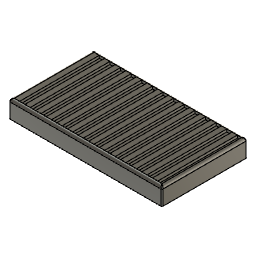
IFEI Clear 0.5mm-0.25 F4 v1 (Autodesk Fusion 360 design; units mm, degrees)
Autodesk Fusion 360 part; units mm, degrees
sketch "Sketch1" plane through (0, 0, 0) normal (0, 0, 1) x (1, 0, 0) in component "Clear"
  line L0 (-0.4, -0.5) -> (13.8, -0.5)
  line L1 (13.9, -0.4) -> (13.9, 7.4)
  line L2 (13.8, 7.5) -> (-0.4, 7.5)
  line L3 (-0.5, 7.4) -> (-0.5, -0.4)
  arc A0 (-0.4, 7.5) -> (-0.5, 7.4) centre (-0.4, 7.4) ccw
  arc A1 (-0.5, -0.4) -> (-0.4, -0.5) centre (-0.4, -0.4) ccw
  arc A2 (13.8, -0.5) -> (13.9, -0.4) centre (13.8, -0.4) ccw
  arc A3 (13.9, 7.4) -> (13.8, 7.5) centre (13.8, 7.4) ccw
  dimension "d4" = 0.1
  dimension "d5" = 0.1
  dimension "d6" = 0.1
  dimension "d7" = 0.1
  constraint tangent L2 A0
  constraint tangent L3 A0
  constraint tangent L3 A1
  constraint tangent L0 A1
  constraint tangent L0 A2
  constraint tangent L1 A2
  constraint tangent L2 A3
  constraint tangent L1 A3
  measures "d4" radius of A0
  measures "d5" radius of A1
  measures "d6" radius of A2
  measures "d7" radius of A3
extrude "Extrude1" add sketch "Sketch1" along normal blind 1.9 in component "Clear"
fillet "Fillet1" radius 0.25 1 faces at (4.3333, 4.8333, 1.9) in component "Clear"
sketch "Sketch1 (2)" plane through (0, 0, 1.9) normal (0, 0, 1) x (-1, 0, 0)
  line L0 (-13.65, 0.25) -> (-13.65, -7.25)
  line L1 (-13.65, -7.25) -> (0.25, -7.25)
  line L2 (0.25, -7.25) -> (0.25, 0.25)
  line L3 (0.25, 0.25) -> (-13.65, 0.25)
  line L4 (0.25, -7.25) -> (-0.25, -7.25) construction
  line L5 (-0.25, -7.25) -> (-0.75, -7.25)
  line L6 (-0.75, -7.25) -> (-0.75, 0.25)
  line L7 (-0.75, 0.25) -> (-0.25, 0.25)
  line L8 (-0.25, 0.25) -> (-0.25, -7.25)
  line L9 (-0.75, -7.25) -> (-1.25, -7.25) construction
  line L10 (-1.75, 0.25) -> (-1.25, 0.25)
  line L11 (-1.75, -7.25) -> (-2.25, -7.25) construction
  line L12 (-1.25, 0.25) -> (-1.25, -7.25)
  line L13 (-1.75, -7.25) -> (-1.75, 0.25)
  line L14 (-1.25, -7.25) -> (-1.75, -7.25)
  line L15 (-3.25, -7.25) -> (-3.75, -7.25)
  line L16 (-2.25, 0.25) -> (-2.25, -7.25)
  line L17 (-2.25, -7.25) -> (-2.75, -7.25)
  line L18 (-3.25, 0.25) -> (-3.25, -7.25)
  line L19 (-3.75, -7.25) -> (-3.75, 0.25)
  line L20 (-3.75, -7.25) -> (-4.25, -7.25) construction
  line L21 (-2.75, 0.25) -> (-2.25, 0.25)
  line L22 (-2.75, -7.25) -> (-2.75, 0.25)
  line L23 (-2.75, -7.25) -> (-3.25, -7.25) construction
  line L24 (-3.75, 0.25) -> (-3.25, 0.25)
  line L25 (-6.75, 0.25) -> (-6.25, 0.25)
  line L26 (-5.25, 0.25) -> (-5.25, -7.25)
  line L27 (-7.75, 0.25) -> (-7.25, 0.25)
  line L28 (-5.75, 0.25) -> (-5.25, 0.25)
  line L29 (-5.25, -7.25) -> (-5.75, -7.25)
  line L30 (-6.75, -7.25) -> (-6.75, 0.25)
  line L31 (-4.75, -7.25) -> (-4.75, 0.25)
  line L32 (-4.75, -7.25) -> (-5.25, -7.25) construction
  line L33 (-6.25, 0.25) -> (-6.25, -7.25)
  line L34 (-4.75, 0.25) -> (-4.25, 0.25)
  line L35 (-7.75, -7.25) -> (-8.25, -7.25) construction
  line L36 (-5.75, -7.25) -> (-6.25, -7.25) construction
  line L37 (-4.25, 0.25) -> (-4.25, -7.25)
  line L38 (-5.75, -7.25) -> (-5.75, 0.25)
  line L39 (-7.25, -7.25) -> (-7.75, -7.25)
  line L40 (-6.75, -7.25) -> (-7.25, -7.25) construction
  line L41 (-7.75, -7.25) -> (-7.75, 0.25)
  line L42 (-7.25, 0.25) -> (-7.25, -7.25)
  line L43 (-6.25, -7.25) -> (-6.75, -7.25)
  line L44 (-4.25, -7.25) -> (-4.75, -7.25)
  line L45 (-12.75, 0.25) -> (-12.25, 0.25)
  line L46 (-13.75, 0.25) -> (-13.25, 0.25)
  line L47 (-8.75, -7.25) -> (-8.75, 0.25)
  line L48 (-13.25, 0.25) -> (-13.25, -7.25)
  line L49 (-8.75, 0.25) -> (-8.25, 0.25)
  line L50 (-9.75, -7.25) -> (-10.25, -7.25) construction
  line L51 (-8.25, 0.25) -> (-8.25, -7.25)
  line L52 (-8.25, -7.25) -> (-8.75, -7.25)
  line L53 (-8.75, -7.25) -> (-9.25, -7.25) construction
  line L54 (-9.25, 0.25) -> (-9.25, -7.25)
  line L55 (-10.75, -7.25) -> (-10.75, 0.25)
  line L56 (-10.75, 0.25) -> (-10.25, 0.25)
  line L57 (-10.75, -7.25) -> (-11.25, -7.25) construction
  line L58 (-9.75, 0.25) -> (-9.25, 0.25)
  line L59 (-11.75, 0.25) -> (-11.25, 0.25)
  line L60 (-11.75, -7.25) -> (-12.25, -7.25) construction
  line L61 (-13.25, -7.25) -> (-13.75, -7.25)
  line L62 (-12.25, 0.25) -> (-12.25, -7.25)
  line L63 (-14.75, -7.25) -> (-15.25, -7.25) construction
  line L64 (-13.75, -7.25) -> (-14.25, -7.25) construction
  line L65 (-12.75, -7.25) -> (-13.25, -7.25) construction
  line L66 (-10.25, -7.25) -> (-10.75, -7.25)
  line L67 (-12.25, -7.25) -> (-12.75, -7.25)
  line L68 (-12.75, -7.25) -> (-12.75, 0.25)
  line L69 (-11.25, 0.25) -> (-11.25, -7.25)
  line L70 (-13.75, -7.25) -> (-13.75, 0.25)
  line L71 (-11.75, -7.25) -> (-11.75, 0.25)
  line L72 (-11.25, -7.25) -> (-11.75, -7.25)
  line L73 (-9.75, -7.25) -> (-9.75, 0.25)
  line L74 (-10.25, 0.25) -> (-10.25, -7.25)
  line L75 (-9.25, -7.25) -> (-9.75, -7.25)
  point P0 (-8.25, -7.25)
  dimension "d11" = 0.5
  dimension "d12" = 0.5
  dimension "d13" = 0.5
  dimension "d14" = 0.5
  dimension "d15" = 0.5
  dimension "d16" = 0.5
  dimension "d17" = 0.5
  dimension "d18" = 0.5
  dimension "d19" = 0.5
  dimension "d20" = 0.5
  dimension "d21" = 0.5
  dimension "d22" = 0.5
  dimension "d23" = 0.5
  dimension "d24" = 0.5
  dimension "d25" = 0.5
  dimension "d26" = 0.5
  dimension "d27" = 0.5
  dimension "d28" = 0.5
  dimension "d29" = 0.5
  dimension "d30" = 0.5
  dimension "d31" = 0.5
  dimension "d32" = 0.5
  dimension "d33" = 0.5
  dimension "d34" = 0.5
  dimension "d35" = 0.5
  dimension "d36" = 0.5
  dimension "d37" = 0.5
  dimension "d38" = 0.5
  dimension "d39" = 0.5
  dimension "d41" = 0.5
  constraint coincident L1.end L2.start
  constraint perpendicular L2 L4
  constraint horizontal L5
  constraint vertical L6
  constraint horizontal L7
  constraint vertical L8
  constraint coincident L3 L6.end
  constraint perpendicular L6 L9
  constraint horizontal L14
  constraint vertical L13
  constraint horizontal L10
  constraint vertical L12
  constraint perpendicular L11 L13
  constraint horizontal L17
  constraint vertical L22
  constraint horizontal L21
  constraint vertical L16
  constraint perpendicular L22 L23
  constraint horizontal L15
  constraint vertical L19
  constraint horizontal L24
  constraint vertical L18
  constraint perpendicular L19 L20
  constraint horizontal L44
  constraint vertical L31
  constraint horizontal L34
  constraint vertical L37
  constraint perpendicular L31 L32
  constraint horizontal L29
  constraint vertical L38
  constraint horizontal L28
  constraint vertical L26
  constraint perpendicular L36 L38
  constraint horizontal L43
  constraint vertical L30
  constraint horizontal L25
  constraint vertical L33
  constraint perpendicular L30 L40
  constraint horizontal L39
  constraint vertical L41
  constraint horizontal L27
  constraint vertical L42
  constraint perpendicular L35 L41
  constraint horizontal L52
  constraint vertical L47
  constraint horizontal L49
  constraint vertical L51
  constraint perpendicular L47 L53
  constraint horizontal L75
  constraint vertical L73
  constraint horizontal L58
  constraint vertical L54
  constraint perpendicular L50 L73
  constraint horizontal L66
  constraint vertical L55
  constraint horizontal L56
  constraint vertical L74
  constraint perpendicular L55 L57
  constraint horizontal L72
  constraint vertical L71
  constraint horizontal L59
  constraint vertical L69
  constraint perpendicular L60 L71
  constraint horizontal L67
  constraint vertical L68
  constraint horizontal L45
  constraint vertical L62
  constraint perpendicular L65 L68
  constraint horizontal L61
  constraint vertical L70
  constraint horizontal L46
  constraint vertical L48
  constraint perpendicular L64 L70
  measures "d11" distance of L1.end L4.end
  measures "d12" distance of L4.end L5.end
  measures "d13" distance of L5.end L9.end
  measures "d14" distance of L11.start L9.end
  measures "d15" distance of L11.start L11.end
  measures "d16" distance of L17.end L11.end
  measures "d17" distance of L17.end L15.start
  measures "d18" distance of L15.end L15.start
  measures "d19" distance of L20.end L15.end
  measures "d20" distance of L31.start L20.end
  measures "d21" distance of L31.start L26.end
  measures "d22" distance of L29.end L26.end
  measures "d23" distance of L33.end L29.end
  measures "d24" distance of L33.end L30.start
  measures "d25" distance of L30.start L39.start
  measures "d26" distance of L39.start L35.start
  measures "d27" distance of P0 L35.start
  measures "d28" distance of L47.start P0
  measures "d29" distance of L53.end L47.start
  measures "d30" distance of L53.end L50.start
  measures "d31" distance of L50.start L50.end
  measures "d32" distance of L50.end L55.start
  measures "d33" distance of L57.end L55.start
  measures "d34" distance of L60.start L57.end
  measures "d35" distance of L60.start L60.end
  measures "d36" distance of L60.end L65.start
  measures "d37" distance of L48.end L65.start
  measures "d38" distance of L48.end L61.end
  measures "d39" distance of L61.end L64.end
  measures "d41" distance of L63.end L63.start
extrude "Extrude2" cut sketch "Sketch1 (2)" against normal blind 0.25 contours L0 L1 L3 L46 L48 L61 | L1 L3 L45 L62 L67 L68 | L1 L3 L59 L69 L71 L72 | L1 L3 L55 L56 L66 L74 | L1 L3 L54 L58 L73 L75 | L1 L3 L47 L49 L51 L52 | L1 L3 L27 L39 L41 L42 | L1 L3 L25 L30 L33 L43 | L1 L3 L26 L28 L29 L38 | L1 L3 L31 L34 L37 L44 | L1 L3 L15 L18 L19 L24 | L1 L3 L16 L17 L21 L22 | L1 L3 L10 L12 L13 L14 | L1 L3 L5 L6 L7 L8 in component "Clear"
move_face "OffsetFaces1" offset -0.25 1 faces at (4.3333, 4.8333, 0) in component "Clear"
component "Clear" placed x (1, 0, 0) y (0, 1, 0) z (0, 0, 1) at (0, 0, 0)
